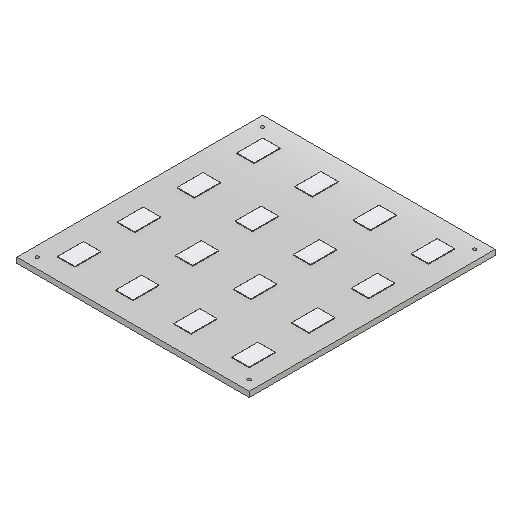
# Autodesk Inventor part: CNCM_ALU_8mm_Thick_Heatbed_Plate
Saved by Autodesk Inventor 2026.1 (Build 301233000, 233)
## iProperties
Created: 2016-06-21
Part Number: CNCM_ALU_8mm_Thick_Heatbed_Plate
Material: Ogólny
Document SubType Name: Modeling
Designer: Andrzej
Density: 1 g/cm^3
Appearance: Obrobione - aluminium
Mass: 788.873 g
Surface Area: 2716.6 cm^2
Volume: 788.873 cm^3
Author: Andrzej
Autodesk Inventor part; units mm, degrees
ref_plane "YZ Plane" through (0, 0, 0) normal (1, 0, 0) x (0, 1, 0)
ref_plane "XZ Plane" through (0, 0, 0) normal (0, 1, 0) x (-1, 0, 0)
ref_plane "XY Plane" through (0, 0, 0) normal (0, 0, 1) x (1, 0, 0)
sketch "Szkic1" plane through (0, 0, 0) normal (0, 0, 1) x (1, 0, 0)
  line L0 (9.4719, 9.8006) -> (352.0719, 9.8006)
  line L1 (352.0719, 9.8006) -> (352.0719, -352.7994)
  line L2 (352.0719, -352.7994) -> (9.4719, -352.7994)
  line L3 (9.4719, -352.7994) -> (9.4719, 9.8006)
  point P0 (0, 0)
  point P1 (24.4719, -337.7994)
  point P2 (337.0719, -337.7994)
  point P3 (24.4719, -5.1994)
  point P4 (337.0719, -5.1994)
  dimension "d0" = 342.6
  dimension "d1" = 362.6
  dimension "d4" = 15
  dimension "d5" = 15
  dimension "d6" = 15
  dimension "d7" = 15
  dimension "d8" = 15
  dimension "d9" = 15
  dimension "d10" = 15
  dimension "d11" = 15
  dimension "d19" = 312.6
  dimension "d20" = 332.6
  constraints: 8 end point, 2 parallel, 1 horizontal, 1 perpendicular
  measures "d0" distance of L1.end L2.end
  measures "d1" distance of L0.end L1.end
  measures "d4" distance from line of point (24.472, -337.799) L2
  measures "d5" distance from line of point (24.472, -337.799) L3
  measures "d6" distance from line of L2 point (337.072, -337.799)
  measures "d7" distance from line of L1 point (337.072, -337.799)
  measures "d8" distance from line of L1 point (337.072, -5.199)
  measures "d9" distance from line of L0 point (337.072, -5.199)
  measures "d10" distance from line of L3 point (24.472, -5.199)
  measures "d11" distance from line of L0 point (24.472, -5.199)
  measures "d19" distance of point (24.472, -5.199) point (337.072, -5.199)
  measures "d20" distance of point (337.072, -337.799) point (337.072, -5.199)
extrude "Wyciągnięcie proste1" add sketch "Szkic1" along normal blind 8
hole "Otwór1" at (24.4719, -337.7994, 0) at (337.0719, -337.7994, 0) at (24.4719, -5.1994, 0) at (337.0719, -5.1994, 0) direction (0, 0, 1) diameter 5 end through all counterbore diameter 10 counterbore depth 4
sketch "Szkic2" plane through (0, 0, 8) normal (0, 0, 1) x (1, 0, 0)
  circle A0 centre (24.4719, -5.1994) radius 2.5 projected
  circle A1 centre (24.4719, -337.7994) radius 2.5 projected
  circle A2 centre (337.0719, -337.7994) radius 2.5 projected
  circle A3 centre (337.0719, -5.1994) radius 2.5 projected
  line L0 (352.0719, 9.8006) -> (9.4719, 9.8006) projected
  line L1 (9.4719, 9.8006) -> (9.4719, -352.7994) projected
  line L2 (9.4719, -352.7994) -> (352.0719, -352.7994) projected
  line L3 (352.0719, -352.7994) -> (352.0719, 9.8006) projected
  line L4 (39.4719, -20.1994) -> (64.9719, -20.1994)
  line L5 (64.9719, -20.1994) -> (64.9719, -58.3994)
  line L6 (64.9719, -58.3994) -> (39.4719, -58.3994)
  line L7 (39.4719, -58.3994) -> (39.4719, -20.1994)
  line L8 (125.1719, -20.1994) -> (150.6719, -20.1994)
  line L9 (150.6719, -20.1994) -> (150.6719, -58.3994)
  line L10 (150.6719, -58.3994) -> (125.1719, -58.3994)
  line L11 (125.1719, -58.3994) -> (125.1719, -20.1994)
  line L12 (210.8719, -20.1994) -> (236.3719, -20.1994)
  line L13 (236.3719, -20.1994) -> (236.3719, -58.3994)
  line L14 (236.3719, -58.3994) -> (210.8719, -58.3994)
  line L15 (210.8719, -58.3994) -> (210.8719, -20.1994)
  line L16 (296.5719, -20.1994) -> (322.0719, -20.1994)
  line L17 (322.0719, -20.1994) -> (322.0719, -58.3994)
  line L18 (322.0719, -58.3994) -> (296.5719, -58.3994)
  line L19 (296.5719, -58.3994) -> (296.5719, -20.1994)
  line L20 (39.4719, -108.3327) -> (64.9719, -108.3327)
  line L21 (64.9719, -108.3327) -> (64.9719, -146.5327)
  line L22 (64.9719, -146.5327) -> (39.4719, -146.5327)
  line L23 (39.4719, -146.5327) -> (39.4719, -108.3327)
  line L24 (125.1719, -108.3327) -> (150.6719, -108.3327)
  line L25 (150.6719, -108.3327) -> (150.6719, -146.5327)
  line L26 (150.6719, -146.5327) -> (125.1719, -146.5327)
  line L27 (125.1719, -146.5327) -> (125.1719, -108.3327)
  line L28 (210.8719, -108.3327) -> (236.3719, -108.3327)
  line L29 (236.3719, -108.3327) -> (236.3719, -146.5327)
  line L30 (236.3719, -146.5327) -> (210.8719, -146.5327)
  line L31 (210.8719, -146.5327) -> (210.8719, -108.3327)
  line L32 (296.5719, -108.3327) -> (322.0719, -108.3327)
  line L33 (322.0719, -108.3327) -> (322.0719, -146.5327)
  line L34 (322.0719, -146.5327) -> (296.5719, -146.5327)
  line L35 (296.5719, -146.5327) -> (296.5719, -108.3327)
  line L36 (39.4719, -196.4661) -> (64.9719, -196.4661)
  line L37 (64.9719, -196.4661) -> (64.9719, -234.6661)
  line L38 (64.9719, -234.6661) -> (39.4719, -234.6661)
  line L39 (39.4719, -234.6661) -> (39.4719, -196.4661)
  line L40 (125.1719, -196.4661) -> (150.6719, -196.4661)
  line L41 (150.6719, -196.4661) -> (150.6719, -234.6661)
  line L42 (150.6719, -234.6661) -> (125.1719, -234.6661)
  line L43 (125.1719, -234.6661) -> (125.1719, -196.4661)
  line L44 (210.8719, -196.4661) -> (236.3719, -196.4661)
  line L45 (236.3719, -196.4661) -> (236.3719, -234.6661)
  line L46 (236.3719, -234.6661) -> (210.8719, -234.6661)
  line L47 (210.8719, -234.6661) -> (210.8719, -196.4661)
  line L48 (296.5719, -196.4661) -> (322.0719, -196.4661)
  line L49 (322.0719, -196.4661) -> (322.0719, -234.6661)
  line L50 (322.0719, -234.6661) -> (296.5719, -234.6661)
  line L51 (296.5719, -234.6661) -> (296.5719, -196.4661)
  line L52 (39.4719, -284.5994) -> (64.9719, -284.5994)
  line L53 (64.9719, -284.5994) -> (64.9719, -322.7994)
  line L54 (64.9719, -322.7994) -> (39.4719, -322.7994)
  line L55 (39.4719, -322.7994) -> (39.4719, -284.5994)
  line L56 (125.1719, -284.5994) -> (150.6719, -284.5994)
  line L57 (150.6719, -284.5994) -> (150.6719, -322.7994)
  line L58 (150.6719, -322.7994) -> (125.1719, -322.7994)
  line L59 (125.1719, -322.7994) -> (125.1719, -284.5994)
  line L60 (210.8719, -284.5994) -> (236.3719, -284.5994)
  line L61 (236.3719, -284.5994) -> (236.3719, -322.7994)
  line L62 (236.3719, -322.7994) -> (210.8719, -322.7994)
  line L63 (210.8719, -322.7994) -> (210.8719, -284.5994)
  line L64 (296.5719, -284.5994) -> (322.0719, -284.5994)
  line L65 (322.0719, -284.5994) -> (322.0719, -322.7994)
  line L66 (322.0719, -322.7994) -> (296.5719, -322.7994)
  line L67 (296.5719, -322.7994) -> (296.5719, -284.5994)
  point P0 (0, 0)
  dimension "d55" = 362.6
  dimension "d56" = 342.6
  dimension "d57" = 30
  dimension "d58" = 30
  dimension "d61" = 85.7
  dimension "d64" = 88.1333
  dimension "d69" = 25.5
  dimension "d70" = 38.2
  constraints: 128 end point, 2 horizontal, 2 parallel, 1 perpendicular, 1 vertical, 120 other
  measures "d55" distance between parallel lines of L2 L0
  measures "d56" distance between parallel lines of L3 L1
  measures "d57" distance between parallel lines of L0 L4
  measures "d58" distance between parallel lines of L1 L7
  measures "d61" distance of L4.start L8.start
  measures "d64" distance of L4.start L20.start
  measures "d69" distance of L5.end L6.end
  measures "d70" distance of L4.end L5.end
extrude "Wyciągnięcie proste2" add sketch "Szkic2" along normal blind 1 contours L4 L5 L6 L7 | L8 L9 L10 L11 | L12 L13 L14 L15 | L16 L17 L18 L19 | L20 L21 L22 L23 | L24 L25 L26 L27 | L28 L29 L30 L31 | L32 L33 L34 L35 | L36 L37 L38 L39 | L40 L41 L42 L43 | L44 L45 L46 L47 | L48 L49 L50 L51 | L52 L53 L54 L55 | L56 L57 L58 L59 | L60 L61 L62 L63 | L64 L65 L66 L67
equation "\"d5\" = d4"
equation "\"d6\" = d4"
equation "\"d7\" = d4"
equation "\"d8\" = d4"
equation "\"d9\" = d4"
equation "\"d10\" = d4"
equation "\"d11\" = d4"
equation "\"d61\" = -0.666667 * d58 + 0.333333 * d56 - 0.333333 * d69"
equation "\"d64\" = -0.666667 * d57 + 0.333333 * d55 - 0.333333 * d70"
